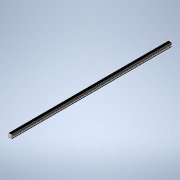
# Autodesk Inventor part: ITEM_20x20_N1_810mm
Saved by Autodesk Inventor 2021 (Build 250183000, 183)
## iProperties
Part Number: ITEM_20x20_N1_810mm
Material: Generic
Document SubType Name: Modeling
Designer: Alexander Fritzsche
Appearance: Default
Author: Alexander Fritzsche
Autodesk Inventor part; units mm, degrees
ref_plane "YZ Plane" through (0, 0, 0) normal (1, 0, 0) x (0, 1, 0)
ref_plane "XZ Plane" through (0, 0, 0) normal (0, 1, 0) x (-1, 0, 0)
ref_plane "XY Plane" through (0, 0, 0) normal (0, 0, 1) x (1, 0, 0)
sketch "Sketch1" plane through (0, 0, 0) normal (0, 0, 1) x (1, 0, 0)
  circle A0 centre (0, 0) radius 2.15
  line L0 (-6.9272, 8.2) -> (-2.3772, 3.65)
  line L1 (-2.3772, 3.65) -> (2.3772, 3.65)
  line L2 (2.3772, 3.65) -> (6.9272, 8.2)
  line L3 (10, 10) -> (10, 2.5)
  line L4 (10, 2.5) -> (8.2, 2.5)
  line L5 (8.2, 2.5) -> (8.2, 6.9272)
  line L6 (8.2, 6.9272) -> (3.65, 2.3772)
  line L7 (3.65, 2.3772) -> (3.65, -2.3772)
  line L8 (3.65, -2.3772) -> (8.2, -6.9272)
  line L9 (8.2, -6.9272) -> (8.2, -2.5)
  line L10 (8.2, -2.5) -> (10, -2.5)
  line L11 (10, -2.5) -> (10, -10)
  line L12 (10, -10) -> (2.5, -10)
  line L13 (2.5, -10) -> (2.5, -8.2)
  line L14 (2.5, -8.2) -> (6.9272, -8.2)
  line L15 (6.9272, -8.2) -> (2.3772, -3.65)
  line L16 (2.3772, -3.65) -> (-2.3772, -3.65)
  line L17 (-2.3772, -3.65) -> (-6.9272, -8.2)
  line L18 (-6.9272, -8.2) -> (-2.5, -8.2)
  line L19 (-2.5, -8.2) -> (-2.5, -10)
  line L20 (-2.5, -10) -> (-10, -10)
  line L21 (-10, -10) -> (-10, -2.5)
  line L22 (-10, -2.5) -> (-8.2, -2.5)
  line L23 (-8.2, -2.5) -> (-8.2, -6.9272)
  line L24 (-8.2, -6.9272) -> (-3.65, -2.3772)
  line L25 (-3.65, -2.3772) -> (-3.65, 2.3772)
  line L26 (-3.65, 2.3772) -> (-8.2, 6.9272)
  line L27 (-8.2, 6.9272) -> (-8.2, 2.5)
  line L28 (-8.2, 2.5) -> (-10, 2.5)
  line L29 (-10, 2.5) -> (-10, 10)
  line L30 (0, 0) -> (-30.8654, 30.8654)
  line L31 (0, 0) -> (30.8654, 30.8654)
  line L32 (0, 0) -> (42.5392, 0)
  line L33 (0, 0) -> (0, 44.3419)
  line L34 (-10, 10) -> (10, 10)
  line L35 (-6.9272, 8.2) -> (6.9272, 8.2)
  dimension "d0" = 45
  dimension "d1" = 90
  dimension "Durchmesser_Loch" = 4.3
  dimension "Wandstaerke" = 1.8
  dimension "d3" = 1.8
  dimension "Breite_Schiene" = 5
  dimension "d16" = 1.8
  dimension "Tiefe_Schiene" = 6.35
  dimension "d18" = 20
  dimension "d19" = 1.8
  dimension "d20" = 5
  constraints: 72 end point, 13 point on line, 12 perpendicular, 9 parallel, 6 collinear, 2 horizontal, 2 vertical, 1 centre point, 1 coincident, 8 other
  measures "d0" angle of L31 L32
  measures "d1" angle of L31 L30
  measures "Durchmesser_Loch" diameter of A0
  measures "Wandstaerke" distance between parallel lines of L0 L26
  measures "d3" distance between parallel lines of L17 L24
  measures "Breite_Schiene" distance between parallel lines of L22 L28
  measures "d16" distance between parallel lines of L34 L35
  measures "Tiefe_Schiene" distance between parallel lines of L34 L1
  measures "d18" distance between parallel lines of L12 L34
  measures "d19" distance of L27.end L28.end
  measures "d20" distance between parallel lines of L13 L19
extrude "Extrusion1" add sketch "Sketch1" along normal mid plane 810 contours L32 L7 L8 L9 L10 L11 L12 L13 L14 L15 L16 L17 L18 L19 L20 L21 L22 L23 L24 L25 L26 L27 L28 L29 L30 A0 | A0 L31 L3 L4 L5 L6 L7 L32 | A0 L33 L1 L2 L35 L34 L31 | L30 L34 L33 L35 L0 L1 A0
fillet "Fillet1" radius 2 4 edges at (10, 10, 0) (-10, 10, 0) (10, -10, 0) (-10, -10, 0)
fillet "Fillet2" radius 0.2 4 edges at (8.2, 2.5, 0) (8.2, -2.5, 0) (-2.5, -8.2, 0) (-8.2, -2.5, 0)
fillet "Fillet3" radius 0.7 14 edges at (10, 2.5, 0) (10, -2.5, 0) (2.5, -10, 0) (-2.5, -10, 0) (-10, -2.5, 0) (-10, 2.5, 0) (-6.9272, -8.2, 0) (-8.2, -6.9272, 0) (6.9272, -8.2, 0) (8.2, -6.9272, 0) (8.2, 6.9272, 0) (-8.2, 6.9272, 0) (-6.9272, 8.2, 0) (6.9272, 8.2, 0)
fillet "Fillet4" radius 2 8 edges at (-3.65, 2.3772, 0) (3.65, 2.3772, 0) (3.65, -2.3772, 0) (2.3772, -3.65, 0) (-2.3772, -3.65, 0) (-3.65, -2.3772, 0) (-2.3772, 3.65, 0) (2.3772, 3.65, 0)
equation "\"d3\" = Wandstaerke"
equation "\"d16\" = Wandstaerke"
equation "\"d19\" = Wandstaerke"
equation "\"d20\" = Breite_Schiene"
body "Solid1"
